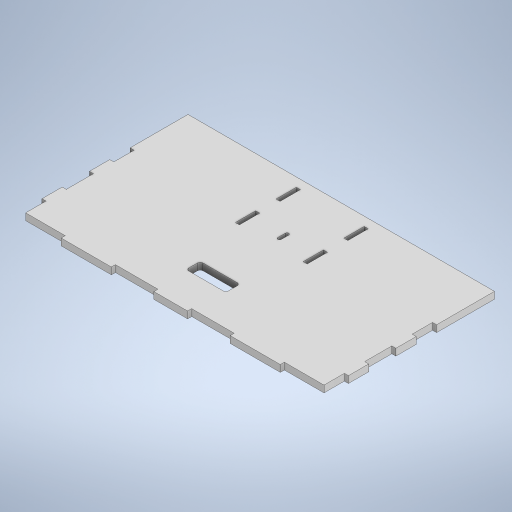
# Autodesk Inventor part: mieng_mat_5mm
Saved by Autodesk Inventor 2023 (Build 270158000, 158)
## iProperties
Created: 2022-11-20
Part Number: mieng_mat_5mm
Material: Generic
Document SubType Name: Modeling
Designer: ADMIN
Density: 1 g/cm^3
Appearance: Default
Author: ADMIN
Autodesk Inventor part; units mm, degrees
ref_plane "YZ Plane" through (0, 0, 0) normal (1, 0, 0) x (0, 1, 0)
ref_plane "XZ Plane" through (0, 0, 0) normal (0, 1, 0) x (-1, 0, 0)
ref_plane "XY Plane" through (0, 0, 0) normal (0, 0, 1) x (1, 0, 0)
sketch "Sketch1" plane through (0, 0, 0) normal (0, 1, 0) x (-1, 0, 0)
  line L0 (16.7044, -242.8336) -> (16.7044, -237.8336)
  line L1 (-20.3174, -242.8336) -> (-20.3174, -237.8336)
  line L2 (-51.677, -242.8336) -> (-51.677, -237.8336)
  line L3 (-76.5581, -242.8336) -> (-76.5581, -237.8336)
  line L4 (-107.9177, -242.8336) -> (-107.9177, -237.8336)
  line L5 (-144.9395, -242.8336) -> (-144.9395, -237.8336)
  line L6 (-174.1176, -242.8336) -> (-144.9395, -242.8336)
  line L7 (-107.9177, -242.8336) -> (-76.5581, -242.8336)
  line L8 (-51.677, -242.8336) -> (-20.3174, -242.8336)
  line L9 (16.7044, -242.8336) -> (45.8824, -242.8336)
  line L10 (48.8824, -272.8336) -> (45.8824, -272.8336)
  line L11 (48.8824, -257.8336) -> (48.8824, -272.8336)
  line L12 (48.8824, -257.8336) -> (45.8824, -257.8336)
  line L13 (45.8824, -292.8336) -> (45.8824, -272.8336)
  line L14 (48.8824, -292.8336) -> (45.8824, -292.8336)
  line L15 (45.8824, -322.8336) -> (45.8824, -307.8336)
  line L16 (48.8824, -307.8336) -> (45.8824, -307.8336)
  line L17 (48.8824, -292.8336) -> (48.8824, -307.8336)
  line L18 (-174.1176, -307.8336) -> (-174.1176, -322.8336)
  line L19 (-177.1176, -307.8336) -> (-174.1176, -307.8336)
  line L20 (-177.1176, -292.8336) -> (-177.1176, -307.8336)
  line L21 (-174.1176, -272.8336) -> (-174.1176, -292.8336)
  line L22 (-177.1176, -292.8336) -> (-174.1176, -292.8336)
  line L23 (-177.1176, -272.8336) -> (-174.1176, -272.8336)
  line L24 (-177.1176, -257.8336) -> (-177.1176, -272.8336)
  line L25 (-177.1176, -257.8336) -> (-174.1176, -257.8336)
  line L26 (-174.1176, -242.8336) -> (-174.1176, -257.8336)
  line L27 (45.8824, -257.8336) -> (45.8824, -242.8336)
  line L28 (16.7044, -239.8336) -> (-20.3174, -239.8336)
  line L29 (-51.677, -239.8336) -> (-76.5581, -239.8336)
  line L30 (-107.9177, -239.8336) -> (-144.9395, -239.8336)
  line L31 (-90.6176, -358.9385) -> (-90.6176, -343.9385)
  line L32 (-90.6176, -343.9385) -> (-87.6176, -343.9385)
  line L33 (-87.6176, -328.9385) -> (-90.6176, -328.9385)
  line L34 (-87.6176, -328.9385) -> (-87.6176, -313.9385)
  line L35 (-87.6176, -313.9385) -> (-90.6176, -313.9385)
  line L36 (-87.6176, -343.9385) -> (-87.6176, -358.9385)
  line L37 (-90.6176, -313.9385) -> (-90.6176, -328.9385)
  line L38 (-90.6176, -343.9385) -> (-90.6176, -358.9385)
  line L39 (-37.6176, -358.9385) -> (-37.6176, -343.9385)
  line L40 (-37.6176, -343.9385) -> (-40.6176, -343.9385)
  line L41 (-40.6176, -328.9385) -> (-40.6176, -313.9385)
  line L42 (-40.6176, -313.9385) -> (-37.6176, -313.9385)
  line L43 (-40.6176, -343.9385) -> (-40.6176, -358.9385)
  line L44 (-37.6176, -313.9385) -> (-37.6176, -328.9385)
  line L45 (-37.6176, -343.9385) -> (-37.6176, -358.9385)
  line L46 (-37.6176, -328.9385) -> (-40.6176, -328.9385)
  line L47 (-37.6176, -358.9385) -> (-40.6176, -358.9385)
  line L48 (-87.6176, -358.9385) -> (-90.6176, -358.9385)
  line L49 (-37.6176, -365.5347) -> (-90.6176, -365.5347)
  line L50 (-37.6176, -365.5347) -> (48.8824, -365.5347)
  line L51 (48.8824, -365.5347) -> (48.8824, -322.8336)
  line L52 (48.8824, -322.8336) -> (45.8824, -322.8336)
  line L53 (-174.1176, -322.8336) -> (-177.1176, -322.8336)
  line L54 (-177.1176, -322.8336) -> (-177.1176, -365.5347)
  line L55 (-177.1176, -365.5347) -> (-90.6176, -365.5347)
  line L56 (-76.7722, -265.7854) -> (-51.4629, -265.7854)
  line L57 (-49.4629, -267.7854) -> (-49.4629, -274.2261)
  line L58 (-51.4629, -276.2261) -> (-76.7722, -276.2261)
  line L59 (-78.7722, -274.2261) -> (-78.7722, -267.7854)
  line L60 (-78.7722, -265.7854) -> (-49.4629, -276.2261) construction
  line L61 (-49.4629, -265.7854) -> (-78.7722, -276.2261) construction
  arc A0 (-51.4629, -276.2261) -> (-49.4629, -274.2261) centre (-51.4629, -274.2261) ccw
  arc A1 (-49.4629, -267.7854) -> (-51.4629, -265.7854) centre (-51.4629, -267.7854) ccw
  arc A2 (-78.7722, -274.2261) -> (-76.7722, -276.2261) centre (-76.7722, -274.2261) ccw
  arc A3 (-76.7722, -265.7854) -> (-78.7722, -267.7854) centre (-76.7722, -267.7854) ccw
  line L62 (-64.1176, -276.2261) -> (-64.1176, -335.7366)
  line L63 (-50.0487, -322.8336) -> (-82.0895, -322.8336)
  line L64 (-62.8676, -320.0836) -> (-62.8676, -325.5836)
  line L65 (-65.3676, -325.5836) -> (-65.3676, -320.0836)
  line L66 (-65.3676, -320.0836) -> (-62.8676, -325.5836) construction
  line L67 (-62.8676, -320.0836) -> (-64.9395, -324.6418) construction
  arc A4 (-65.3676, -325.5836) -> (-62.8676, -325.5836) centre (-64.1176, -325.5836) ccw
  arc A5 (-62.8676, -320.0836) -> (-65.3676, -320.0836) centre (-64.1176, -320.0836) ccw
  point P0 (0, 0)
  point P1 (-126.4286, -237.8336)
  point P2 (-177.1176, -300.3336)
  point P3 (48.8824, -300.3336)
  point P4 (-35.9972, -242.8336)
  point P5 (-64.1176, -271.0058)
  point P6 (-64.1176, -322.8336)
  dimension "d2" = 5
  dimension "d3" = 15
  dimension "d4" = 15
  dimension "d5" = 20
  dimension "d6" = 15
  dimension "d7" = 15
  dimension "d8" = 220
  dimension "d9" = 226
  dimension "d10" = 31.3596
  dimension "d11" = 37.0218
  dimension "d12" = 29.178
  dimension "d13" = 24.8811
  dimension "d14" = 31.3596
  dimension "d15" = 37.0218
  dimension "d16" = 29.178
  dimension "d17" = 15
  dimension "d18" = 15
  dimension "d19" = 20
  dimension "d20" = 15
  dimension "d21" = 15
  dimension "d27" = 15
  dimension "d28" = 3
  dimension "d30" = 15
  dimension "d31" = 122.7011
  dimension "d32" = 2
  dimension "d33" = 80
  dimension "d34" = 2.5
  dimension "d35" = 5.5
  constraints: 136 end point, 21 point on line, 12 point on circle, 9 perpendicular, 8 horizontal, 8 tangent, 7 midpoint, 6 centre point, 4 vertical, 3 equal radius, 3 parallel, 2 collinear
  measures "d2" distance of L0.start L0.end
  measures "d3" distance of L11.start L11.end
  measures "d4" distance of L27.start L27.end
  measures "d5" distance of L14.end L10.end
  measures "d6" distance of L14.start L17.end
  measures "d7" distance of L15.start L16.end
  measures "d8" distance of L18.end L15.start
  measures "d9" distance of point (-177.118, -300.334) point (48.882, -300.334)
  measures "d10" distance of L2.start L1.start
  measures "d11" distance of L1.end L0.end
  measures "d12" distance of L0.start L27.end
  measures "d13" distance of L3.end L2.end
  measures "d14" distance of L4.start L7.end
  measures "d15" distance of L5.end L4.end
  measures "d16" distance of L6.start L5.start
  measures "d17" distance of L6.start L26.end
  measures "d18" distance of L25.start L24.end
  measures "d19" distance of L23.end L21.end
  measures "d20" distance of L22.start L20.end
  measures "d21" distance of L19.end L18.end
  measures "d27" distance of L31.start L31.end
  measures "d28" distance of L31.end L32.end
  measures "d30" distance of L33.start L34.end
  measures "d31" distance from line of point (-35.997, -242.834) L50
  measures "d32" radius of A0
  measures "d33" distance between parallel lines of L63 L8
  measures "d34" distance of L65.start L64.end
  measures "d35" distance of L64.end L64.start
extrude "Extrusion1" add sketch "Sketch1" along normal blind 5
body "Solid1"
